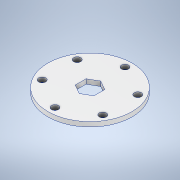
# Autodesk Inventor part: InnerHexHub
Saved by Autodesk Inventor 2020 (Build 240168000, 168)
## iProperties
Created: 2019-06-06
Part Number: InnerHexHub
Material: Aluminum 6061
Document SubType Name: Modeling
Designer: Connor
Density: 2.7 g/cm^3
Appearance: Aluminum - Flat
Author: Connor
Autodesk Inventor part; units mm, degrees
ref_plane "YZ Plane" through (0, 0, 0) normal (1, 0, 0) x (0, 1, 0)
ref_plane "XZ Plane" through (0, 0, 0) normal (0, 1, 0) x (-1, 0, 0)
ref_plane "XY Plane" through (0, 0, 0) normal (0, 0, 1) x (1, 0, 0)
sketch "Sketch1" plane through (0, 0, 0) normal (0, 1, 0) x (-1, 0, 0)
  line L0 (0, -7.3323) -> (-6.35, -3.6662)
  line L1 (-6.35, -3.6662) -> (-6.35, 3.6662)
  line L2 (-6.35, 3.6662) -> (0, 7.3323)
  line L3 (0, 7.3323) -> (6.35, 3.6662)
  line L4 (6.35, 3.6662) -> (6.35, -3.6662)
  line L5 (6.35, -3.6662) -> (0, -7.3323)
  circle A0 centre (0, 0) radius 28.575
  dimension "d0" = 12.7
  dimension "d2" = 57.15
  constraints: 12 end point, 2 coincident, 1 centre point, 1 vertical alignment, 13 other
  measures "d0" distance between parallel lines of L1 L4
  measures "d2" diameter of A0
extrude "Extrusion1" add sketch "Sketch1" along normal blind 3.175
sketch "Sketch2" plane through (0, 3.175, 0) normal (0, 1, 0) x (1, 0, 0)
  point P0 (0, 0)
  point P1 (0, 23.8125)
  point P2 (-20.6222, 11.9063)
  point P3 (-20.6222, -11.9062)
  point P4 (0, -23.8125)
  point P5 (20.6222, -11.9063)
  point P6 (20.6222, 11.9062)
  dimension "d5" = 23.8125
  dimension "d8" = 360
  constraints: 1 vertical alignment, 7 other
  measures "d5" distance of point (0, 0) point (0, 23.812)
hole "Hole1" at (0, 3.175, -23.8125) at (-20.6222, 3.175, -11.9063) at (-20.6222, 3.175, 11.9062) at (0, 3.175, 23.8125) at (20.6222, 3.175, 11.9063) at (20.6222, 3.175, -11.9062) direction (0, -1, 0) diameter 4.826 end through all
sketch "Sketch3" plane through (0, 3.175, 0) normal (0, 1, 0) x (1, 0, 0)
  circle A0 centre (20.6222, -11.9063) radius 2.413 projected
  circle A1 centre (-20.6222, -11.9062) radius 2.413 projected
  circle A2 centre (0, 23.8125) radius 2.413 projected
  circle A3 centre (-20.6222, 11.9063) radius 2.413 projected
  circle A4 centre (0, -23.8125) radius 2.413 projected
  circle A5 centre (20.6222, 11.9062) radius 2.413 projected
  circle A6 centre (0, 0) radius 28.575 projected
  line L0 (0, -7.3323) -> (-6.35, -3.6662) projected
  line L1 (-6.35, -3.6662) -> (-6.35, 3.6662) projected
  line L2 (-6.35, 3.6662) -> (0, 7.3323) projected
  line L3 (0, 7.3323) -> (6.35, 3.6662) projected
  line L4 (6.35, 3.6662) -> (6.35, -3.6662) projected
  line L5 (6.35, -3.6662) -> (0, -7.3323) projected
  circle A7 centre (0, 23.8125) radius 5.588 construction
  circle A8 centre (20.6222, 11.9062) radius 5.588 construction
  circle A9 centre (20.6222, -11.9063) radius 5.588 construction
  circle A10 centre (0, -23.8125) radius 5.588 construction
  circle A11 centre (-20.6222, -11.9062) radius 5.588 construction
  circle A12 centre (-20.6222, 11.9063) radius 5.588 construction
  circle A13 centre (-11.1563, 19.3233) radius 6.4377 construction
  circle A14 centre (11.1563, 19.3233) radius 6.4377 construction
  circle A15 centre (11.1563, -19.3233) radius 6.4377 construction
  circle A16 centre (-11.1563, -19.3233) radius 6.4377 construction
  circle A17 centre (-22.3127, 0) radius 6.4377 construction
  circle A18 centre (22.3127, 0) radius 6.4377 construction
  circle A19 centre (0, 0) radius 15.875 construction
  arc A20 (-16.2237, 15.3528) -> (-21.4077, 6.3737) centre (-20.6222, 11.9063) ccw
  arc A21 (-21.4077, -6.3737) -> (-21.4077, 6.3737) centre (-22.3127, 0) ccw
  circle A22 centre (-20.6222, -11.9062) radius 2.413 projected
  arc A23 (-21.4077, -6.3737) -> (-16.2237, -15.3528) centre (-20.6222, -11.9062) ccw
  arc A24 (-5.184, -21.7265) -> (-16.2237, -15.3528) centre (-11.1563, -19.3233) ccw
  arc A25 (-5.184, -21.7265) -> (5.184, -21.7265) centre (0, -23.8125) ccw
  arc A26 (16.2237, -15.3528) -> (5.184, -21.7265) centre (11.1563, -19.3233) ccw
  arc A27 (16.2237, -15.3528) -> (21.4077, -6.3737) centre (20.6222, -11.9063) ccw
  arc A28 (21.4077, 6.3737) -> (21.4077, -6.3737) centre (22.3127, 0) ccw
  arc A29 (21.4077, 6.3737) -> (16.2237, 15.3528) centre (20.6222, 11.9062) ccw
  arc A30 (5.184, 21.7265) -> (16.2237, 15.3528) centre (11.1563, 19.3233) ccw
  arc A31 (5.184, 21.7265) -> (-5.184, 21.7265) centre (0, 23.8125) ccw
  arc A32 (-16.2237, 15.3528) -> (-5.184, 21.7265) centre (-11.1563, 19.3233) ccw
  dimension "d19" = 3.175
  dimension "d20" = 31.75
  constraints: 48 point on circle, 25 centre point, 19 coincident, 18 tangent, 5 equal radius
  measures "d19" radial gap between concentric circles of A7 A2
  measures "d20" diameter of A19
extrude "Extrusion2" [suppressed]
body "Solid1"
